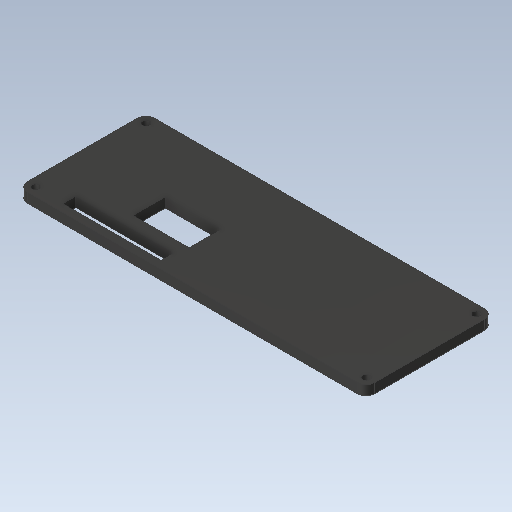
# Autodesk Inventor part: 5_pokrywa wyświetlacza
Saved by Autodesk Inventor 2020.2 (Build 242310000, 310)
## iProperties
Created: 2017-10-07
Part Number: 5_pokrywa wyświetlacza
Material: Ogólny
Document SubType Name: Modeling
Designer: Haras2
Density: 1 g/cm^3
Appearance: Domyślna
Author: Haras2
Autodesk Inventor part; units mm, degrees
ref_plane "YZ Plane" through (0, 0, 0) normal (1, 0, 0) x (0, 1, 0)
ref_plane "XZ Plane" through (0, 0, 0) normal (0, 1, 0) x (-1, 0, 0)
ref_plane "XY Plane" through (0, 0, 0) normal (0, 0, 1) x (1, 0, 0)
sketch "Szkic1" plane through (0, 0, 0) normal (0, 1, 0) x (-1, 0, 0)
  line L0 (0, 0) -> (-161, 0)
  line L1 (-161, 0) -> (-161, -59)
  line L2 (-161, -59) -> (0, -59)
  line L3 (0, -59) -> (0, 0)
  dimension "d0" = 161
  dimension "d1" = 59
  constraints: 11 end point, 2 parallel, 1 coincident, 1 horizontal, 1 perpendicular
  measures "d0" distance of L0.start L0.end
  measures "d1" distance of L0.start L2.end
extrude "Wyciągnięcie proste1" add sketch "Szkic1" along normal blind 4.5
sketch "Szkic2" plane through (0, 4.5, 0) normal (0, 1, 0) x (1, 0, 0)
  line L0 (38, 30) -> (64, 30)
  line L1 (64, 30) -> (64, 15)
  line L2 (64, 15) -> (38, 15)
  line L3 (38, 15) -> (38, 30)
  line L4 (17, 9.5) -> (62.5, 9.5)
  line L5 (62.5, 9.5) -> (62.5, 3.5)
  line L6 (62.5, 3.5) -> (17, 3.5)
  line L7 (17, 3.5) -> (17, 9.5)
  line L8 (0, 0) -> (161, 0) projected
  line L9 (0, 59) -> (0, 0) projected
  dimension "d15" = 26
  dimension "d16" = 15
  dimension "d17" = 6
  dimension "d18" = 45.5
  dimension "d19" = 3.5
  dimension "d20" = 15
  dimension "d21" = 17
  dimension "d22" = 38
  constraints: 16 end point, 4 parallel, 2 horizontal, 2 perpendicular
  measures "d15" distance between parallel lines of L1 L3
  measures "d16" distance of L0.end L1.end
  measures "d17" distance of L4.end L5.end
  measures "d18" distance between parallel lines of L7 L5
  measures "d19" distance between parallel lines of L8 L6
  measures "d20" distance between parallel lines of L8 L2
  measures "d21" distance between parallel lines of L9 L7
  measures "d22" distance between parallel lines of L9 L3
extrude "Wyciągnięcie proste2" cut sketch "Szkic2" against normal through all
sketch "Szkic3" plane through (0, 4.5, 0) normal (0, 1, 0) x (1, 0, 0)
  line L0 (161, 59) -> (0, 59) projected
  line L1 (161, 0) -> (161, 59) projected
  point P0 (0, 0)
  point P1 (4, 55)
  point P2 (4, 4)
  point P3 (157, 55)
  point P4 (157, 4)
  dimension "d25" = 51
  dimension "d26" = 153
  dimension "d27" = 4
  dimension "d28" = 4
  constraints: 2 horizontal alignment, 2 vertical alignment
  measures "d25" distance of point (4, 4) point (4, 55)
  measures "d26" distance of point (157, 4) point (4, 4)
  measures "d27" distance from line of L0 point (4, 55)
  measures "d28" distance from line of L1 point (157, 4)
hole "Otwór1" at (4, 4.5, -55) at (4, 4.5, -4) at (157, 4.5, -55) at (157, 4.5, -4) direction (0, -1, 0) diameter 3.5 end through all
fillet "Zaokrąglenie1" radius 4 4 edges at (0, 2.25, -59) (0, 2.25, 0) (161, 2.25, -59) (161, 2.25, 0)
